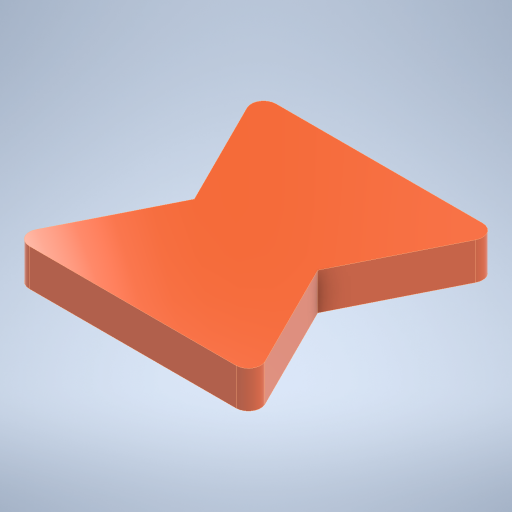
# Autodesk Inventor part: Test2
Saved by Autodesk Inventor 2023.1 (Build 271208000, 208)
## iProperties
Created: 2023-02-07
Part Number: Test2
Material: ABS Plastic
Document SubType Name: Modeling
Designer: 19644
Density: 1.06 g/cm^3
Appearance: Smooth - Light Orange
Author: 19644
## iProperties of the stored document Test2_3DPrint.ipt
Created: 2023-02-07
Part Number: Test2_3DPrint
Material: Generic
Document SubType Name: Modeling
Designer: 19644
Density: 1 g/cm^3
Appearance: Default
Author: 19644
Autodesk Inventor part; units mm, degrees
ref_plane "YZ Plane" through (0, 0, 0) normal (1, 0, 0) x (0, 1, 0)
ref_plane "XZ Plane" through (0, 0, 0) normal (0, 1, 0) x (-1, 0, 0)
ref_plane "XY Plane" through (0, 0, 0) normal (0, 0, 1) x (1, 0, 0)
sketch "Sketch1" plane through (0, 0, 0) normal (0, 1, 0) x (-1, 0, 0)
  line L0 (20.6295, 20.0875) -> (-19.3705, 20.0875)
  line L1 (20.6295, 20.0875) -> (10.6295, 0.0875)
  line L2 (-19.3705, 20.0875) -> (-9.3705, 0.0875)
  line L3 (20.6295, -19.9125) -> (-19.3705, -19.9125)
  line L4 (20.6295, -19.9125) -> (10.6295, 0.0875)
  line L5 (-19.3705, -19.9125) -> (-9.3705, 0.0875)
  dimension "d12" = 40
  dimension "d27" = 40
  dimension "d34" = 20
  dimension "d35" = 20
  dimension "d36" = 20
  dimension "d38" = 10
  constraints: 12 end point, 1 horizontal
  measures "d12" distance of L0.start L0.end
  measures "d27" distance of L4.start L3.end
  measures "d34" distance of L2.end L1.end
  measures "d35" distance from line of L2.end L3
  measures "d36" distance from line of L0 L2.end
  measures "d38" horizontal distance of L0.end L2.end
extrude "Extrusion8" add sketch "Sketch1" along normal blind 6
fillet "Fillet4" radius 2 4 edges at (-20.6295, 3, 20.0875) (19.3705, 3, 20.0875) (19.3705, 3, -19.9125) (-20.6295, 3, -19.9125)
body "Solid5"
